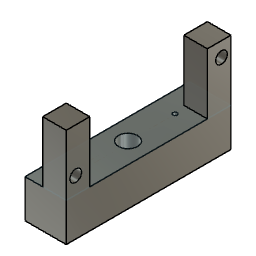
servo 1 bracket (Autodesk Fusion 360 design; units mm, degrees)
Autodesk Fusion 360 part; units mm, degrees
sketch "Sketch1" plane through (0, 0, 0) normal (0, 0, 1) x (1, 0, 0)
  line L0 (7, -22) -> (-7, -22)
  line L1 (-7, -22) -> (-7, 22)
  line L2 (-7, 22) -> (7, 22)
  line L3 (7, 22) -> (7, -22)
  line L4 (7, -22) -> (-7, 22) construction
  line L5 (-7, -22) -> (7, 22) construction
  circle A0 centre (0, 0) radius 3.2483
  circle A1 centre (0, 16) radius 0.75
  circle A2 centre (0, -16) radius 0.75
  dimension "d1" = 1.5
  dimension "d2" = 1.5
  constraint horizontal L0
  constraint perpendicular L0 L1
  constraint parallel L0 L2
  constraint parallel L1 L3
  constraint coincident L4 A0.centre
  constraint coincident L5 A0.centre
  constraint coincident A0.centre origin
  measures "d1" diameter of A1
  measures "d2" diameter of A2
extrude "Extrude1" add sketch "Sketch1" along normal blind 13
extrude "Extrude2" add 1 faces at (-2.3333, 22, 4.3333) along direction (0, 1, 0) blind 6
extrude "Extrude3" add 1 faces at (2.3333, -22, 4.3333) along direction (0, -1, 0) blind 6
sketch "Sketch2" plane through (0, 0, 13) normal (0, 0, 1) x (-1, 0, 0)
  circle A0 centre (0, 0) radius 3.2483
  circle A1 centre (0, 16) radius 0.75
  circle A2 centre (0, -16) radius 0.75
  line L0 (7, -28) -> (7, 28)
  line L1 (7, 28) -> (-7, 28)
  line L2 (-7, 28) -> (-7, -28)
  line L3 (-7, -28) -> (7, -28)
sketch "Sketch3" plane through (0, 0, 13) normal (0, 0, 1) x (-1, 0, 0)
  line L0 (7, -28) -> (-7, -28)
  line L1 (-7, -28) -> (-7, -20)
  line L2 (-7, -20) -> (7, -20)
  line L3 (7, -20) -> (7, -28)
  line L4 (7, 20) -> (-7, 20)
  line L5 (-7, 20) -> (-7, 28)
  line L6 (-7, 28) -> (7, 28)
  line L7 (7, 28) -> (7, 20)
  constraint horizontal L0
  constraint vertical L1
  constraint horizontal L2
  constraint vertical L3
  constraint horizontal L4
  constraint vertical L5
  constraint horizontal L6
  constraint vertical L7
extrude "Extrude4" add sketch "Sketch3" along normal blind 11
extrude "Extrude5" add 2 faces at (-2.3333, 25.3333, 24) (-2.3333, -22.6667, 24) along direction (0, 0, 1) blind 9.65
sketch "Sketch4" plane through (7, 0, 0) normal (1, 0, 0) x (0, 1, 0)
  line L0 (-28, 0) -> (28, 0)
  line L1 (28, 0) -> (28, 33.65)
  line L2 (28, 33.65) -> (20, 33.65)
  line L3 (20, 33.65) -> (20, 13)
  line L4 (20, 13) -> (-20, 13)
  line L5 (-20, 13) -> (-20, 33.65)
  line L6 (-20, 33.65) -> (-28, 33.65)
  line L7 (-28, 33.65) -> (-28, 0)
  circle A0 centre (-24.7678, 18.6815) radius 2.0007
  circle A1 centre (24.8, 28.7) radius 2.0005
  dimension "d13" = 4.001
  measures "d13" diameter of A1
extrude "Extrude6" cut sketch "Sketch4" against normal blind 15 contours A0 | A1
sketch "Sketch5" plane through (-7, 0, 0) normal (-1, 0, 0) x (0, -1, 0)
  circle A0 centre (24.7678, 18.6815) radius 2.0007
  circle A1 centre (-24.8, 28.7) radius 2.0005
  line L0 (-28, 0) -> (28, 0)
  line L1 (28, 0) -> (28, 33.65)
  line L2 (28, 33.65) -> (20, 33.65)
  line L3 (20, 33.65) -> (20, 13)
  line L4 (20, 13) -> (-20, 13)
  line L5 (-20, 13) -> (-20, 33.65)
  line L6 (-20, 33.65) -> (-28, 33.65)
  line L7 (-28, 33.65) -> (-28, 0)
  line L8 (-28, 13) -> (28, 13)
  line L9 (28, 13) -> (28, 35.3728)
  line L10 (28, 35.3728) -> (-28, 35.3728)
  line L11 (-28, 35.3728) -> (-28, 13)
  constraint horizontal L8
  constraint vertical L9
  constraint horizontal L10
  constraint vertical L11
  constraint coincident L7 L8.start
extrude "Extrude7" cut sketch "Sketch5" against normal blind 6 contours L5 L6 L7 L8 L11 | L1 L2 L3 L8 L9
extrude "Extrude8" [suppressed]
extrude "Extrude9" [suppressed]
extrude "Extrude10" [suppressed]
extrude "Extrude11" [suppressed]
